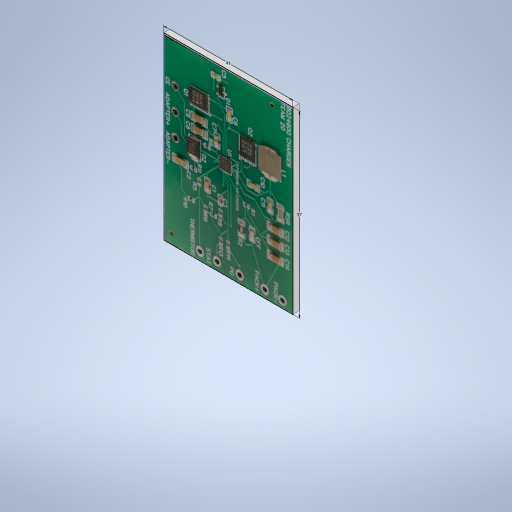
# Autodesk Inventor part: BQ24600 PCB Mockup
Saved by Autodesk Inventor 2023 (Build 270158000, 158)
## iProperties
Created: 2023-04-23
Part Number: BQ24600 PCB Mockup
Material: Generic
Document SubType Name: Modeling
Designer: ethan
Density: 1 g/cm^3
Appearance: Default
Author: ethan
Autodesk Inventor part; units mm, degrees
ref_plane "YZ Plane" through (0, 0, 0) normal (1, 0, 0) x (0, 1, 0)
ref_plane "XZ Plane" through (0, 0, 0) normal (0, 1, 0) x (-1, 0, 0)
ref_plane "XY Plane" through (0, 0, 0) normal (0, 0, 1) x (1, 0, 0)
sketch "Sketch1" plane through (0, 0, 0) normal (0, 0, 1) x (1, 0, 0)
  line L0 (0, 0) -> (41, 0)
  line L1 (41, 0) -> (41, 57)
  line L2 (41, 57) -> (0, 57)
  line L3 (0, 57) -> (0, 0)
  line L4 (40.9471, 56.5933) -> (40.9471, -0.0129) construction
  line L5 (40.9471, -0.0129) -> (0.1741, -0.0129) construction
  line L6 (0.1741, -0.0129) -> (0.1741, 56.5933) construction
  line L7 (0.1741, 56.5933) -> (40.9471, 56.5933) construction
  dimension "d0" = 41
  dimension "d1" = 57
  constraints: 8 end point, 2 parallel, 1 horizontal, 1 perpendicular, 2 other
  measures "d0" distance of L2.end L1.end
  measures "d1" distance of L1.end L0.end
extrude "Extrusion2" add sketch "Sketch1" against normal blind 2
body "Solid2"
